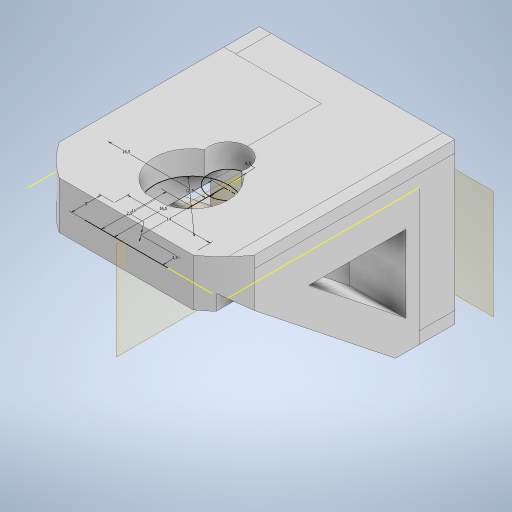
# Autodesk Inventor part: roka3
Saved by Autodesk Inventor 2024 (Build 280153000, 153)
## iProperties
Created: 2023-09-03
Part Number: roka3
Material: Generic
Document SubType Name: Modeling
Designer: jebes windows
Density: 1 g/cm^3
Appearance: Default
Author: jebes windows
## iProperties of the stored document roka3_3DPrint.ipt
Created: 2023-09-09
Part Number: roka3_3DPrint
Material: Generic
Document SubType Name: Modeling
Designer: jebes windows
Density: 1 g/cm^3
Appearance: Default
Author: jebes windows
Autodesk Inventor part; units mm, degrees
ref_plane "YZ Plane" through (0, 0, 0) normal (1, 0, 0) x (0, 1, 0)
ref_plane "XZ Plane" through (0, 0, 0) normal (0, 1, 0) x (-1, 0, 0)
ref_plane "XY Plane" through (0, 0, 0) normal (0, 0, 1) x (1, 0, 0)
ref_plane "Work Plane1" through (0, 0, 0) normal (0, 0, 1) x (1, 0, 0)
sketch "Sketch1" plane through (0, 0, 0) normal (0, 0, 1) x (1, 0, 0)
  line L0 (1.899876, -6.449999) -> (1.899874, -2.879669)
  arc A0 (1.899874, -2.879669) -> (2.208946, -2.649998) centre (-0.000127, 0.000001) ccw
  line L1 (2.208946, -2.649998) -> (14.158996, -1.997015)
  arc A1 (14.158996, -1.997015) -> (14.158994, 1.997027) centre (14.049873, 0.000006) ccw
  line L2 (14.158994, 1.997027) -> (2.208944, 2.650002)
  arc A2 (2.208944, 2.650002) -> (1.899872, 2.879672) centre (-0.000127, 0.000001) ccw
  line L3 (1.899872, 2.879672) -> (1.899871, 6.450001)
  arc A3 (1.899871, 6.450001) -> (-1.900129, 6.45) centre (-0.000129, 6.450001) ccw
  line L4 (-1.900129, 6.45) -> (-1.900128, 3.29535)
  line L5 (-1.900128, 3.29535) -> (-16.626419, 1.99221)
  arc A4 (-16.626419, 1.99221) -> (-16.626418, -1.992221) centre (-16.450127, -0.000005) ccw
  line L6 (-16.626418, -1.992221) -> (-1.900126, -3.29535)
  line L7 (-1.900126, -3.29535) -> (-1.900124, -6.45)
  arc A5 (-1.900124, -6.45) -> (1.899876, -6.449999) centre (-0.000124, -6.449999) ccw
  circle A6 centre (-14.850127, -0.000005) radius 0.6
  circle A7 centre (-16.850127, -0.000006) radius 0.6
  circle A8 centre (-12.850127, -0.000004) radius 0.6
  circle A9 centre (-10.850127, -0.000003) radius 0.6
  circle A10 centre (-8.850127, -0.000003) radius 0.6
  circle A11 centre (-6.850127, -0.000002) radius 0.6
  circle A12 centre (-4.850127, -0.000001) radius 0.6
  circle A13 centre (4.449873, 0.000002) radius 0.6
  circle A14 centre (6.449873, 0.000003) radius 0.6
  circle A15 centre (8.449873, 0.000004) radius 0.6
  circle A16 centre (10.449873, 0.000005) radius 0.6
  circle A17 centre (14.449873, 0.000006) radius 0.6
  circle A18 centre (12.449873, 0.000005) radius 0.6
  circle A19 centre (-0.000127, 0.000001) radius 2.3
  circle A20 centre (-0.000125, -4.449999) radius 0.6
  circle A21 centre (-0.000124, -6.449999) radius 0.6
  circle A22 centre (-0.000128, 4.450001) radius 0.6
  circle A23 centre (-0.000129, 6.450001) radius 0.6
  arc A24 (-5.155188, -3.137951) -> (-5.155065, 3.138505) centre (0.249873, 0.000171) ccw
  arc A25 (-5.155065, 3.138505) -> (-5.155188, -3.137951) centre (-6.000127, 0.000294) ccw
  line L8 (-19.750353, -11.499436) -> (-19.749901, 11.500564)
  line L9 (9.249647, -11.500006) -> (-19.750353, -11.499436)
  line L10 (9.250099, 11.499994) -> (9.249647, -11.500006)
  line L11 (-19.749901, 11.500564) -> (9.250099, 11.499994)
  line L12 (-21.749901, 11.500603) -> (-21.750353, -11.499397)
  line L13 (11.249647, -11.500045) -> (11.250099, 11.499955)
  line L14 (-19.750392, -13.499436) -> (9.249608, -13.500006)
  line L15 (9.250138, 13.499994) -> (-19.749862, 13.500564)
  line L16 (9.249608, -13.500006) -> (11.249647, -13.500006)
  line L17 (11.249647, -13.500006) -> (11.249647, -11.500045)
  line L18 (11.250099, 11.499955) -> (11.250099, 13.499994)
  line L19 (9.250138, 13.499994) -> (11.250099, 13.499994)
  line L20 (-19.749862, 13.500564) -> (-21.749901, 13.500564)
  line L21 (-21.749901, 11.500603) -> (-21.749901, 13.500564)
  line L22 (-21.750353, -11.499397) -> (-21.750353, -13.499436)
  line L23 (-21.750353, -13.499436) -> (-19.750392, -13.499436)
  point P0 (0, 0)
  constraints: 16 end point, 4 horizontal, 4 vertical
extrude "Extrusion1" add sketch "Sketch1" along normal blind 6 contours A5 L7 A24 A21 L0 | L0 A24 L1 L10 L9 L8 L11 L2 L3 A3 L4 A25 L5 A4 L6 L7 A5 | A24 A21 L7 L6 A25 A10 L5 L4 A23 L3 A2 L2 A14 L1 A0 L0 | L0 A0 L1 A24 | A24 A21 | A21 A24 | A24 A14 L2 L10 L1 | A24 A25 L6 L7 | L10 L2 L13 L1 | L1 L13 L17 L16 L14 L23 L22 L12 L21 L20 L15 L19 L18 L2 L10 L11 L8 L9 | L6 A4 L5 A25 A10 | L2 A2 L3 A24 | A25 A10 | A10 A25 | A24 A23 L4 A3 L3 | A24 A23 | A23 A24 | A25 A24 L4 L5 | A6 | A7 | A8 | A9 | A15 | A16 | A20 | A22
sketch "Sketch10" plane through (0, 0, 6) normal (0, 0, 1) x (1, 0, 0)
  line L0 (11.250099, 11.499955) -> (11.250099, 13.499994)
  line L1 (11.250099, 13.499994) -> (9.250138, 13.499994)
  line L2 (9.250138, 13.499994) -> (-19.749862, 13.500564)
  line L3 (-19.749862, 13.500564) -> (-21.749901, 13.500564)
  line L4 (-21.749901, 13.500564) -> (-21.749901, 11.500603)
  line L5 (-21.749901, 11.500603) -> (-21.750353, -11.499397)
  line L6 (-21.750353, -11.499397) -> (-21.750353, -13.499436)
  line L7 (-21.750353, -13.499436) -> (-19.750392, -13.499436)
  line L8 (-19.750392, -13.499436) -> (9.249608, -13.500006)
  line L9 (9.249608, -13.500006) -> (11.249647, -13.500006)
  line L10 (11.249647, -13.500006) -> (11.249647, -11.500045)
  line L11 (11.249647, -11.500045) -> (11.250099, 11.499955)
  line L12 (-19.749862, 13.500564) -> (-21.749901, 13.500564)
  line L13 (-21.749901, 13.500564) -> (-21.74994, 9.500564)
  line L14 (-21.749901, 11.500603) -> (-21.750353, -11.499397)
  line L15 (-21.74994, 9.500564) -> (11.25006, 9.499916)
  line L16 (11.249647, -11.500045) -> (11.250099, 11.499955)
  line L17 (11.250099, 13.499994) -> (11.25006, 9.499916)
  line L18 (11.250099, 11.499955) -> (11.250099, 13.499994)
  line L19 (11.250099, 13.499994) -> (-21.749901, 13.500564)
  point P0 (0, 0)
  point P1 (-5.249577, 13.500279)
  point P2 (11.25006, 9.499916)
  dimension "d42" = 4
  constraints: 8 end point, 2 point on line, 1 perpendicular
  measures "d42" distance of L3.end L13.end
extrude "Extrusion7" add sketch "Sketch10" along normal blind 33 contours L11 L15 L5 L4 L3 L2 L1 L0
sketch "Sketch11" plane through (11.25006, 9.499916, 6) normal (-0.0000196, -1, 0) x (1, -0.0000196, 0)
  line L0 (0, 0) -> (-33, 0)
  line L1 (-16.499715, 0) -> (-16.499715, 33)
  line L2 (-2, 33) -> (-16.499715, 33)
  line L3 (-16.499715, 33) -> (-16.499715, 22)
  circle A0 centre (-16.499715, 22) radius 6.25
  circle A1 centre (-16.499715, 15.75) radius 3.25
  line L4 (-9.5, 33) -> (-23.5, 33)
  line L5 (-23.5, 33) -> (-23.5, 28)
  line L6 (-23.5, 28) -> (-9.5, 28)
  line L7 (-9.5, 28) -> (-9.5, 33)
  line L8 (-9.5, 33) -> (-23.5, 28) construction
  line L9 (-23.5, 33) -> (-9.5, 28) construction
  line L10 (-33, 0) -> (-33, 33)
  circle A2 centre (-16.5, 30.5) radius 1.25
  line L11 (-16.499715, 33) -> (-16.499715, 16.5)
  line L12 (-16.499715, 16.5) -> (0, 16.5)
  line L13 (0, 0) -> (0, 33)
  line L14 (-9.5, 0) -> (-23.5, 0)
  line L15 (-23.5, 0) -> (-23.5, 5)
  line L16 (-23.5, 5) -> (-9.5, 5)
  line L17 (-9.5, 5) -> (-9.5, 0)
  line L18 (-9.5, 0) -> (-23.5, 5) construction
  line L19 (-23.5, 0) -> (-9.5, 5) construction
  circle A3 centre (-16.5, 2.5) radius 1.25
  point P0 (-11.249873, -6)
  point P1 (-23.5, 0)
  point P2 (-9.5, 0)
  point P3 (-18.249715, 28)
  point P4 (-14.749715, 28)
  point P5 (-9.5, 33)
  point P6 (-19.637943, 16.595)
  point P7 (-13.337438, 16.5)
  point P8 (-13.53113, 16.5)
  dimension "d47" = 12.5
  dimension "d46" = 11
  dimension "d48" = 6.5
  dimension "d49" = 14
  dimension "d50" = 5
  dimension "d51" = 2.5
  dimension "d52" = 16.5
  dimension "d53" = 2.5
  dimension "d54" = 16.5
  constraints: 30 end point, 6 symmetric about line, 4 midpoint, 3 centre point, 3 coincident, 2 parallel, 2 point on line, 1 horizontal, 1 perpendicular, 4 other
  measures "d46" distance of L1.end L3.end
  measures "d48" diameter of A1
  measures "d49" distance of L6.end L5.end
  measures "d50" distance of L5.end L4.end
  measures "d51" distance from line of L2 point (-16.5, 30.5)
  measures "d52" distance from line of L10 point (-16.5, 30.5)
  measures "d53" diameter of A2
  measures "d54" distance of L1.end L11.end
extrude "Extrusion9" cut sketch "Sketch11" against normal through all contours A1 L1 A0 L12 | A1 L1 L6 A0 | A0 L12 L1 A1 | A0 L1 L12 | A1 A0 L1 | A1 A0 L6 L1 | L1 A0 A1
extrude "Extrusion8" add sketch "Sketch11" along normal blind 4 contours L0 L1 A3 L16 L17 | L0 L15 L16 L1 A3 | L6 L1 A0 | A0 L1 A2 L2 L7 L6 | L6 L5 L4 L1 A2 A0 | A0 L1 L6
sketch "Sketch12" plane through (-21.74994, 9.500564, 6) normal (-0.0000196, -1, 0) x (1, -0.0000196, 0)
  line L0 (32.999961, -6) -> (32.999961, 33)
  line L1 (32.999961, 33) -> (29.999961, 33)
  line L2 (32.999961, 33) -> (31, 33)
  line L3 (29.999961, 33) -> (29.999961, -6)
  line L4 (31, -6) -> (2, -6)
  line L5 (32.999961, -6) -> (31, -6)
  line L6 (32.999961, 33) -> (32.999961, -6)
  line L7 (-0.000039, 0) -> (-0.000039, 33)
  line L8 (-0.000039, 33) -> (2.999961, 33)
  line L9 (16.500285, 33) -> (-0.000039, 33)
  line L10 (2.999961, 33) -> (2.999961, -6)
  line L11 (2, -6) -> (-0.000039, -6)
  line L12 (2.999961, -6) -> (-0.000039, -6)
  line L13 (-0.000039, -6) -> (-0.000039, 0)
  line L14 (-0.000039, -6) -> (-0.000039, 33)
  point P0 (21.750127, -6)
  dimension "d59" = 3
  dimension "d60" = 3
  constraints: 14 end point, 3 point on line, 2 collinear, 2 perpendicular, 1 horizontal, 1 vertical
  measures "d59" distance of L0.end L1.end
  measures "d60" distance of L7.end L8.end
extrude "Extrusion10" add sketch "Sketch12" along normal up to surface (22.999961 mm away)
sketch "Sketch13" plane through (-21.749979, 9.500564, 0) normal (-1, 0.0000196, 0) x (0, 0, 1)
  line L0 (0, -22.999961) -> (39, -22.999961)
  line L1 (39, 0) -> (39, -22.999961)
  line L2 (39, 0) -> (0, 0)
  line L3 (0, 0) -> (0, -22.999961)
  line L4 (0, 0) -> (39, 0)
  line L5 (0, -22.999921) -> (0, -20.999961)
  line L6 (0, 0) -> (0, -22.999921)
  line L7 (0, -22.999921) -> (10, -22.999961)
  line L8 (10, -22.999961) -> (39, 0)
  line L9 (24.649218, -5) -> (5, -5)
  line L10 (5, -5) -> (5, -17.999941)
  line L11 (5, -17.999941) -> (8.257943, -17.999954)
  line L12 (8.257943, -17.999954) -> (24.649218, -5)
  line L13 (8.257943, -17.999954) -> (8.257943, -5)
  dimension "d89" = 10
  dimension "d90" = 5
  constraints: 18 end point, 2 collinear, 2 point on line, 1 perpendicular, 3 other
  measures "d89" distance of L5.start L7.end
  measures "d90" distance between parallel lines of L8 L12
extrude "Extrusion11" cut sketch "Sketch13" against normal blind 4 contours L8 L1 L0 | L12 L13 L9
ref_plane "Work Plane3" through (-5.249979, 9.50024, 39) normal (1, -0.0000196, 0) x (0, 0, -1)
mirror "Mirror3" about plane through (-5.249979, 9.50024, 39) normal (1, -0.0000196, 0) of "Extrusion11"
sketch "Sketch15" plane through (-12.24994, 9.500377, 6) normal (-0.0000196, -1, 0) x (1, -0.0000196, 0)
  line L0 (-6.500039, 33) -> (-6.500039, 0)
  line L1 (0, 0) -> (-6.500039, 0)
  line L2 (0, 0) -> (0, 5)
  line L3 (0, 5) -> (14, 5)
  line L4 (14, 5) -> (14, 0)
  line L5 (20.499961, 0) -> (14, 0)
  line L6 (20.499961, 0) -> (20.499961, 33)
  line L7 (14, 33) -> (20.499961, 33)
  line L8 (14, 33) -> (14, 28)
  line L9 (14, 28) -> (8.750285, 28)
  arc A0 (9.96887, 16.5) -> (8.750285, 28) centre (7.000285, 22) ccw
  line L10 (9.96887, 16.5) -> (10.162562, 16.5)
  arc A1 (3.862057, 16.595) -> (10.162562, 16.5) centre (7.000285, 15.75) ccw
  arc A2 (5.250285, 28) -> (3.862057, 16.595) centre (7.000285, 22) ccw
  line L11 (5.250285, 28) -> (0, 28)
  line L12 (0, 28) -> (0, 33)
  line L13 (-6.500039, 33) -> (0, 33)
  line L14 (0, 28) -> (0, 5)
  line L15 (14, 28) -> (14, 5)
  point P0 (12.250127, -6)
  constraints: 4 end point, 1 collinear, 1 vertical
extrude "Extrusion12" add sketch "Sketch15" along normal up to surface (22.999961 mm away) contours L13 L12 L14 L2 L1 L0 | L15 L8 L7 L6 L5 L4
sketch "Sketch16" plane through (-18.750078, 4.500505, 8.257943) normal (-1, 0.0000196, 0) x (0, 0, 1)
  line L0 (16.391274, 0) -> (0, 0)
  line L1 (0, 0) -> (0, -12.999954)
  line L2 (0, -12.999954) -> (16.391274, 0)
  line L3 (30.742057, 5) -> (1.742057, -17.999961)
  line L4 (1.742057, -17.999961) -> (30.742057, -17.999961)
  line L5 (30.742057, 5) -> (30.742057, -17.999961)
  line L6 (30.742057, 1) -> (30.742057, -17.999961)
  line L7 (30.742057, 1) -> (25.69857, 1)
  line L8 (25.742057, 1) -> (30.742057, 1)
  point P0 (-8.257943, -4.500137)
  constraints: 2 end point, 1 collinear, 1 point on line
extrude "Extrusion13" cut sketch "Sketch16" against normal through all contours L2 L1 L0 | L7 L5 L4 L3
sketch "Sketch18" plane through (-5.249577, 13.500279, 18.5) normal (0.0000173, 1, 0) x (1, -0.0000173, 0)
  line L0 (16.499676, 18.5) -> (16.499676, -20.5)
  line L1 (14.499715, -20.5) -> (0, -20.5)
  line L2 (0, -20.5) -> (-16.500324, -20.5)
  circle A0 centre (-0.000307, -4.000017) radius 16.499983
  circle A1 centre (-0.000307, -4.000017) radius 20
  line L3 (16.499676, -20.5) -> (14.499715, -20.5)
  line L4 (-16.500324, 12.5) -> (-16.500324, -20.5)
  line L5 (-16.500324, 18.5) -> (-16.500324, 12.5)
  line L6 (14.499715, 18.5) -> (-14.500285, 18.5)
  point P0 (5.24981, 18.5)
  point P1 (16.499676, 17.5)
  point P2 (16.499676, -15.302697)
  point P3 (11.302373, -20.5)
  point P4 (-16.500324, -15.302647)
  point P5 (-11.302987, -20.5)
  dimension "d111" = 40
  dimension "d112" = 22.50002
  constraints: 2 centre point, 2 tangent, 1 coincident
  measures "d111" diameter of A1
  measures "d112" distance from line of L6 A0.centre
extrude "Extrusion15" cut sketch "Sketch18" against normal through all contours L0 L3 L1 A1 | A1 L2 L4
body "Solid1"
